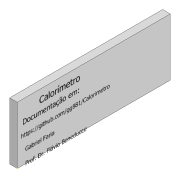
# Autodesk Inventor part: Placa
Saved by Autodesk Inventor 2020 (Build 240168000, 168)
## iProperties
Created: 2022-08-02
Part Number: Placa
Material: Genérico
Document SubType Name: Modeling
Designer: gabri
Density: 1 g/cm^3
Appearance: Padrão
Author: gabri
Autodesk Inventor part; units mm, degrees
ref_plane "YZ Plane" through (0, 0, 0) normal (1, 0, 0) x (0, 1, 0)
ref_plane "XZ Plane" through (0, 0, 0) normal (0, 1, 0) x (-1, 0, 0)
ref_plane "XY Plane" through (0, 0, 0) normal (0, 0, 1) x (1, 0, 0)
sketch "Esboço1" plane through (0, 0, 0) normal (1, 0, 0) x (0, 1, 0)
  line L0 (0, 0) -> (30, 0)
  line L1 (30, 0) -> (30, -80)
  line L2 (30, -80) -> (0, -80)
  line L3 (0, -80) -> (0, 0)
  dimension "d0" = 80
  dimension "d1" = 30
  constraints: 8 end point, 2 parallel, 1 horizontal, 1 perpendicular
  measures "d0" distance of L2.end L0.start
  measures "d1" distance of L1.end L2.end
extrude "Extrusão1" add sketch "Esboço1" along normal blind 4
sketch "Esboço2" plane through (4, 0, 0) normal (1, 0, 0) x (0, 0, -1)
  line L0 (11.4929, 26.8754) -> (32.8289, 26.8754) construction
  line L1 (32.8289, 26.8754) -> (32.8289, 23.3803) construction
  line L2 (32.8289, 23.3803) -> (11.4929, 23.3803) construction
  line L3 (11.4929, 23.3803) -> (11.4929, 26.8754) construction
  line L4 (2.6931, 20.997) -> (38.2588, 20.997) construction
  line L5 (38.2588, 20.997) -> (38.2588, 12.2889) construction
  line L6 (38.2588, 12.2889) -> (2.6931, 12.2889) construction
  line L7 (2.6931, 12.2889) -> (2.6931, 20.997) construction
  line L8 (1.9598, 14.4889) -> (40.4587, 14.4889) construction
  line L9 (40.4587, 14.4889) -> (40.4587, 10.5473) construction
  line L10 (40.4587, 10.5473) -> (1.9598, 10.5473) construction
  line L11 (1.9598, 10.5473) -> (1.9598, 14.4889) construction
  line L12 (4.1598, 7.7974) -> (41.192, 7.7974) construction
  line L13 (41.192, 7.7974) -> (41.192, 2.1142) construction
  line L14 (41.192, 2.1142) -> (4.1598, 2.1142) construction
  line L15 (4.1598, 2.1142) -> (4.1598, 7.7974) construction
  point P0 (0, 0)
  constraints: 8 other
